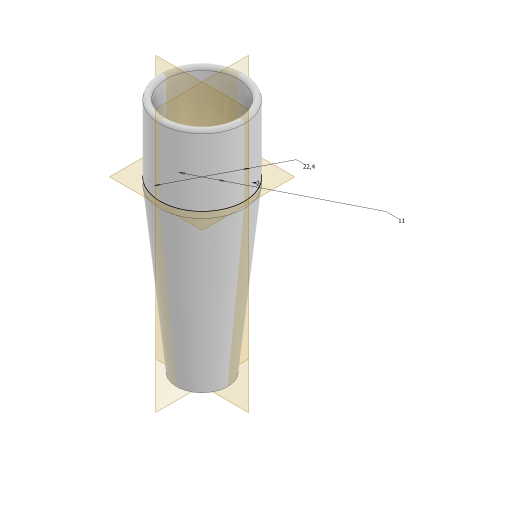
# Autodesk Inventor part: Стакан для крепления ходовой гайки
Saved by Autodesk Inventor 2023.2 (Build 272271030, 271C)
## iProperties
Created: 2025-04-10
Part Number: Стакан для крепления ходовой гайки
Material: Типовые
Document SubType Name: Modeling
Designer: Коноваленко
Density: 1 g/cm^3
Appearance: По умолчанию
Author: Коноваленко
Autodesk Inventor part; units mm, degrees
sketch "Эскиз1" plane through (0, 0, 0) normal (0, 1, 0) x (-1, 0, 0)
  circle A0 centre (0, 0) radius 11.2
  circle A1 centre (0, 0) radius 13.2
  circle A2 centre (0, 0) radius 5.5
  dimension "d0" = 22.4
  dimension "d1" = 2
  dimension "d2" = 11
  constraints: 3 centre point, 3 coincident
  measures "d0" diameter of A0
  measures "d1" radial gap between concentric circles of A1 A0
  measures "d2" diameter of A2
extrude "Выдавливание1" add sketch "Эскиз1" along normal blind 22 contours A1
extrude "Выдавливание2" add sketch "Эскиз1" against normal blind 2 contours A0 | A1
fillet "Сопряжение1" radius 1 2 edges at (13.2, 22, 0) (11.2, 22, 0)
sketch "Эскиз2" plane through (0, 0, 0) normal (1, 0, 0) x (0, 1, 0)
  line L0 (-53, 0) -> (-53, -8)
  line L1 (-53, 0) -> (-2, 0)
  line L2 (-69.0693, 0) -> (-63.203, 0)
  line L3 (-2, 13.2) -> (-2, -13.2)
  line L4 (-2, 13.2) -> (-2, -13.2) projected
  line L5 (-53, -8) -> (-2, -13.2)
  point P0 (0, 0)
  dimension "d13" = 51
  dimension "d14" = 8
  constraints: 10 end point, 1 horizontal, 1 vertical
  measures "d13" distance of L0.start L1.end
  measures "d14" distance of L0.start L0.end
revolve "Вращение1" add sketch "Эскиз2" angle 360 about axis through (0, -69.0693, 0) along (0, 1, 0)
extrude "Выдавливание3" cut sketch "Эскиз1" against normal up to surface (53 mm away) contours A2
sketch "Эскиз5" plane through (0, -53, 0) normal (0, -1, 0) x (1, 0, 0)
  circle A0 centre (0, 0) radius 5.15
  circle A1 centre (0, 0) radius 5.5 projected
  dimension "d18" = 10.3
  constraints: 1 centre point, 1 coincident
  measures "d18" diameter of A0
extrude "Выдавливание4" add sketch "Эскиз5" against normal blind 46
